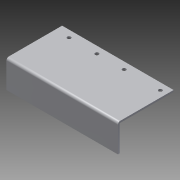
# Autodesk Inventor part: Electrical Board Mount Part1
Saved by Autodesk Inventor 2013 (Build 170138000, 138)
## iProperties
Created: 2013-01-26
Part Number: Electrical Board Mount Part1
Material: Aluminum 6061
Document SubType Name: Sheet Metal
Designer: Moses
Density: 2.71 g/cm^3
Sheet Metal Rule: Default
Mass: 152.68 g
Surface Area: 723.123 cm^2
Volume: 56.3394 cm^3
Author: Moses
Autodesk Inventor part; units mm, degrees
ref_plane "YZ Plane" through (0, 0, 0) normal (1, 0, 0) x (0, 1, 0)
ref_plane "XZ Plane" through (0, 0, 0) normal (0, 1, 0) x (-1, 0, 0)
ref_plane "XY Plane" through (0, 0, 0) normal (0, 0, 1) x (1, 0, 0)
sketch "Sketch1" plane through (0, 0, 0) normal (0, 1, 0) x (-1, 0, 0)
  line L0 (0, 0) -> (203.2, 0)
  line L1 (203.2, 0) -> (203.2, 25.4)
  line L2 (203.2, 25.4) -> (0, 25.4) construction
  line L3 (0, 25.4) -> (0, 0)
  line L4 (11.45, 12.7) -> (77.45, 12.7) construction
  circle A0 centre (11.45, 12.7) radius 3.302
  circle A1 centre (77.45, 12.7) radius 3.302
  line L5 (44.45, 25.4) -> (44.45, 0) construction
  circle A2 centre (127, 12.7) radius 3.302
  circle A3 centre (177.8, 12.7) radius 3.302
  line L6 (127, 12.7) -> (177.8, 12.7) construction
  line L7 (152.4, 25.4) -> (152.4, 0) construction
  line L8 (0, 25.4) -> (0, 101.6)
  line L9 (0, 101.6) -> (203.2, 101.6)
  line L10 (203.2, 101.6) -> (203.2, 25.4)
  point P0 (44.45, 12.7)
  point P1 (152.4, 12.7)
  dimension "d0" = 66
  dimension "d1" = 6.604
  dimension "d2" = 6.604
  dimension "d3" = 25.4
  dimension "d4" = 44.45
  dimension "d6" = 50.8
  dimension "d7" = 50.8
  dimension "d8" = 76.2
  dimension "d9" = 203.2
  measures "d0" distance of L4.start L4.end
  measures "d1" diameter of A0
  measures "d2" diameter of A1
  measures "d3" distance of L2.end L0.start
  measures "d4" distance between parallel lines of L5 L3
  measures "d6" distance of L6.end L6.start
  measures "d7" distance between parallel lines of L1 L7
  measures "d8" distance of L2.end L8.end
  measures "d9" distance of L8.end L9.end
extrude "Plate1" add sketch "Sketch1" along normal blind 3.175
sketch "Sketch2" plane through (-203.2, 3.175, 98.425) normal (0, 0, 1) x (1, 0, 0)
  line L0 (203.2, 0) -> (0, 0)
  line L1 (0, 0) -> (0, -50.8)
  line L2 (0, -50.8) -> (203.2, -50.8)
  line L3 (203.2, -50.8) -> (203.2, 0)
  constraints: 6 end point, 1 horizontal, 1 perpendicular, 1 vertical
edge flange "Flange1" height 50.8 angle 90 thickness 3.175 bend radius 1.27 thickness toward (0, 0, 1) relief tear relief width 3.175 relief depth 1.5875 edges at (-101.6, 0, 101.6) wall of the first edge with corners at (0, 3.175, 98.425) (-203.2, 3.175, 98.425) (-203.2, -47.625, 98.425) (0, -47.625, 98.425)
bend "Bend1"
corner "Corner1"
equation "\"d11\" = BendReliefWidth"
equation "\"d12\" = BendReliefDepth"
equation "\"d13\" = MinimumRemnant"
equation "\"d14\" = BendRadius"
equation "\"d18\" = CornerReliefSize"
equation "\"d19\" = GapSize"
equation "\"d20\" = JacobiRadiusSize"
equation "\"BendRadius\" = Thickness"
equation "\"BendReliefWidth\" = Thickness"
equation "\"BendReliefDepth\" = 0.5 * Thickness"
equation "\"CornerReliefSize\" = 4 * Thickness"
equation "\"MinimumRemnant\" = 2 * Thickness"
equation "\"TransitionRadius\" = BendRadius"
equation "\"JacobiRadiusSize\" = BendRadius"
equation "\"GapSize\" = Thickness"
equation "\"d10\" = BendRadius"
equation "\"Thickness\" = 3.175"
body "Solid1"
